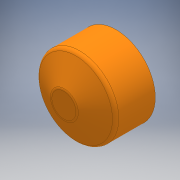
# Autodesk Inventor part: paris_pivot_cup
Saved by Autodesk Inventor 2019 (Build 230136000, 136)
## iProperties
Created: 2017-04-02
Part Number: paris_pivot_cup
Material: Типовые
Document SubType Name: Modeling
Designer: Nikita
Density: 1 g/cm^3
Appearance: Оранжевый
Author: Nikita
Autodesk Inventor part; units mm, degrees
ref_plane "YZ Plane" through (0, 0, 0) normal (1, 0, 0) x (0, 1, 0)
ref_plane "XZ Plane" through (0, 0, 0) normal (0, 1, 0) x (-1, 0, 0)
ref_plane "XY Plane" through (0, 0, 0) normal (0, 0, 1) x (1, 0, 0)
sketch "Эскиз1" plane through (0, 0, 0) normal (0, 0, 1) x (1, 0, 0)
  line L0 (0, 0) -> (3, 0)
  line L1 (3, 0) -> (9, 3)
  line L2 (9, 3) -> (9, 12)
  line L3 (9, 12) -> (6.5, 12)
  line L4 (6.5, 12) -> (6.5, 7)
  line L5 (0, 2) -> (0, 0)
  line L6 (0, 2) -> (1.5, 2)
  arc A0 (1.5, 2) -> (6.5, 7) centre (1.5, 7) ccw
  dimension "d0" = 18
  dimension "d2" = 13
  dimension "d3" = 12
  dimension "d4" = 9
  dimension "d5" = 6
  dimension "d6" = 10
  dimension "d9" = 1.5
  dimension "d10" = 5
  constraints: 14 end point, 3 perpendicular, 2 horizontal, 2 point on circle, 1 centre point, 1 tangent, 1 vertical
  measures "d0" diameter of L2 L5
  measures "d2" diameter of L4 L5
  measures "d3" distance between parallel lines of L0 L3
  measures "d4" distance of L1.end L2.end
  measures "d5" diameter of L0.end L5
  measures "d6" distance from line of L5.start L3
  measures "d9" distance of L5.start L6.end
  measures "d10" radius of A0
revolve "Вращение1" add sketch "Эскиз1" angle 360 about axis through (0, 2, 0) along (0, -1, 0)
fillet "Сопряжение1" radius 1 2 edges at (-9, 3, 0) (-3, 0, 0)
